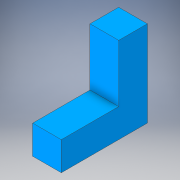
# Autodesk Inventor part: Blue part
Saved by Autodesk Inventor 2017 (Build 210142000, 142)
## iProperties
Created: 2016-11-01
Part Number: Blue part
Material: Generic
Document SubType Name: Modeling
Designer: rbibb
Density: 1 g/cm^3
Appearance: Default
Author: rbibb
Autodesk Inventor part; units mm, degrees
ref_plane "YZ Plane" through (0, 0, 0) normal (1, 0, 0) x (0, 1, 0)
ref_plane "XZ Plane" through (0, 0, 0) normal (0, 1, 0) x (-1, 0, 0)
ref_plane "XY Plane" through (0, 0, 0) normal (0, 0, 1) x (1, 0, 0)
sketch "Sketch1" plane through (0, 0, 0) normal (1, 0, 0) x (0, 1, 0)
  point P0 (0, 0)
sketch "Sketch2" plane through (0, 0, 0) normal (1, 0, 0) x (0, 1, 0)
  line L0 (13.9517, 18.9807) -> (-43.1983, 18.9807)
  line L1 (-43.1983, 18.9807) -> (-43.1983, -0.0693)
  line L2 (-43.1983, -0.0693) -> (13.9517, -0.0693)
  line L3 (13.9517, -0.0693) -> (13.9517, 18.9807)
  point P0 (0, 0)
  dimension "d0" = 57.15
  dimension "d1" = 19.05
  constraints: 8 end point, 2 parallel, 1 horizontal, 1 perpendicular
  measures "d0" distance of L2.end L1.end
  measures "d1" distance of L1.end L0.end
extrude "Extrusion1" add sketch "Sketch2" along normal blind 19.05
sketch "Sketch3" plane through (0, -43.1983, 18.9807) normal (0, 0, 1) x (1, 0, 0)
  line L0 (0, 57.15) -> (0, 0) projected
  line L1 (19.05, 57.15) -> (19.05, 0) projected
  line L2 (0, 0) -> (19.05, 0)
  line L3 (19.05, 0) -> (19.05, 19.05)
  line L4 (19.05, 19.05) -> (0, 19.05)
  line L5 (0, 19.05) -> (0, 0)
  point P0 (0, 43.1983)
  dimension "d4" = 19.05
  constraints: 8 end point, 2 parallel, 1 horizontal, 1 perpendicular, 1 point on line
  measures "d4" distance of L3.end L2.end
extrude "Extrusion2" add sketch "Sketch3" along normal blind 38.1
body "Solid1"
